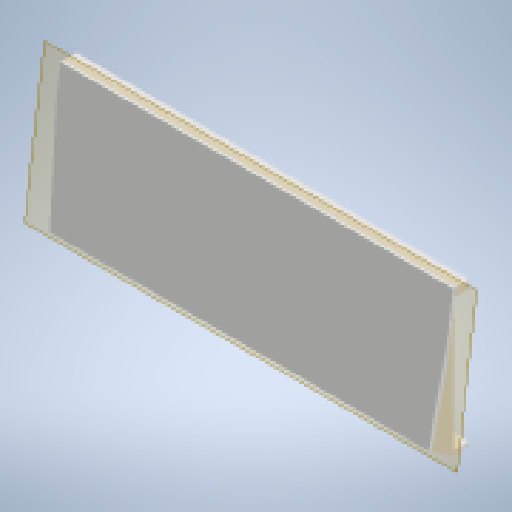
# Autodesk Inventor part: bottom
Saved by Autodesk Inventor 2024.2 (Build 282272000, 272)
## iProperties
Created: 2024-07-29
Part Number: bottom
Material: Generic
Document SubType Name: Modeling
Designer: Eric
Density: 1 g/cm^3
Appearance: Default
Author: Eric
Autodesk Inventor part; units mm, degrees
ref_plane "Work Plane1" through (0, 0, 9.8) normal (0, 0, 1) x (1, 0, 0)
sketch "Sketch1" plane through (0, 0, 9.8) normal (0, 0, 1) x (1, 0, 0)
  line L0 (145.35, 54.1) -> (-145.35, 54.1) projected
  line L1 (145.35, -54.1) -> (145.35, 54.1) projected
  line L2 (-145.35, -54.1) -> (145.35, -54.1) projected
  line L3 (-145.35, 54.1) -> (-145.35, -54.1) projected
  line L4 (143.1, 53.975) -> (-143.1, 53.975)
  line L5 (-143.1, 53.975) -> (-143.1, -51.85)
  line L6 (-143.1, -51.85) -> (143.1, -51.85)
  line L7 (143.1, -51.85) -> (143.1, 53.975)
  point P0 (0, 0)
  dimension "d0" = 0.125
  dimension "d1" = 2.25
  dimension "d2" = 2.25
  dimension "d3" = 2.25
  constraints: 8 end point, 2 parallel, 1 horizontal, 1 perpendicular
  measures "d0" distance between parallel lines of L0 L4
  measures "d1" distance between parallel lines of L2 L6
  measures "d2" distance between parallel lines of L1 L7
  measures "d3" distance between parallel lines of L3 L5
ref_plane "Work Plane2" through (-147.35, 31.7362, 13.0715) normal (0, 0.1305262, 0.9914449) x (1, 0, 0)
extrude "Extrusion1" add sketch "Sketch1" along normal up to surface contours L7 L6 L5 L4 surface through (-147.35, 31.7362, 13.0715) normal (0, 0.1305262, 0.9914449)
sketch "Sketch3" plane through (0, 0, 9.8) normal (0, 0, -1) x (-1, 0, 0)
  line L0 (143.1, 48.1) -> (-143.1, 48.1)
  line L1 (-143.1, -51.85) -> (-143.1, 53.975) projected
  line L2 (-143.1, -48.1) -> (143.1, -48.1)
  line L3 (143.1, 53.975) -> (143.1, -51.85) projected
  line L4 (-143.1, 53.975) -> (143.1, 53.975) projected
  line L5 (143.1, -51.85) -> (-143.1, -51.85) projected
  point P0 (0, 0)
  dimension "d8" = 5.875
  dimension "d9" = 3.75
  constraints: 4 end point, 3 point on line, 1 horizontal, 1 parallel
  measures "d8" distance between parallel lines of L4 L0
  measures "d9" distance between parallel lines of L5 L2
ref_plane "Work Plane3" through (-145.35, -54.1, -1.5) normal (0, 0, 1) x (1, 0, 0)
extrude "Extrusion2" add sketch "Sketch3" along normal up to surface (11.3 mm away) contours L0 L1 L4 L3 | L3 L5 L1 L2
sketch "Sketch4" plane through (-143.1, -48.1, 9.8) normal (-1, 0, 0) x (0, 0, 1)
  line L0 (14.2758, -3.75) -> (0.3437, 102.075) projected
  line L1 (13.3027, 3.6417) -> (1.7, -3.75)
  line L2 (-11.3, -3.75) -> (14.2758, -3.75) projected
  line L3 (0.7, -6) -> (0.7, -8) projected
  point P0 (-9.8, 48.1)
  dimension "d12" = 65
  dimension "d23" = 1
  constraints: 2 end point, 2 point on line
  measures "d12" angle of L0 L1
  measures "d23" distance from line of L3 L1.end
extrude "Extrusion3" cut sketch "Sketch4" against normal through all
sketch "Sketch5" plane through (-143.1, -51.85, -1.5) normal (0, -1, 0) x (1, 0, 0)
  line L0 (0, 13) -> (0, 24.6027) projected
  line L1 (0, 13) -> (5.4104, 24.6027)
  line L2 (0, 24.6027) -> (286.2, 24.6027) projected
  point P0 (143.1, 1.5)
  dimension "d15" = 65
  constraints: 2 end point, 1 point on line
  measures "d15" angle of L2 L1
sketch "Sketch6" plane through (-143.1, -48.1, 9.8) normal (-1, 0, 0) x (0, 0, 1)
  line L0 (1.7, -3.75) -> (3.3295, 79.3957)
  point P0 (-9.8, 48.1)
  point P1 (0.3437, 102.075)
  dimension "d16" = 22.875
  constraints: 2 end point
  measures "d16" distance of point (0.344, 102.075) L0.end
sweep "Sweep1" cut profiles "Sketch5" path "Sketch6"
mirror "Mirror1" about plane through (0, 0, 0) normal (1, 0, 0) of "Sweep1"
ref_plane "Work Plane4" through (-143.1, 53.7139, 8.1608) normal (0, 0.1305262, 0.9914449) x (1, 0, 0)
sketch "Sketch8" plane through (-143.1, 53.975, 10.1437) normal (0, 0.1305262, 0.9914449) x (1, 0, 0)
  line L0 (286.2, 0) -> (286.2, -22.875) projected
  line L1 (286.2, -15) -> (0, -15)
  line L2 (0, -22.875) -> (0, 0) projected
  line L3 (0, 0) -> (286.2, 0) projected
  point P0 (143.1, -52.1892)
  dimension "d20" = 15
  constraints: 2 end point, 2 point on line, 1 horizontal
  measures "d20" distance between parallel lines of L3 L1
extrude "Extrusion4" add sketch "Sketch8" against normal up to surface (2 mm away)
sketch "Sketch9" plane through (-143.1, -51.85, -1.5) normal (0, -1, 0) x (1, 0, 0)
  line L0 (286.2, 0) -> (286.2, 11.6437) projected
  line L1 (286.2, 3) -> (0, 3)
  line L2 (0, 10.3999) -> (0, 0) projected
  line L3 (286.2, 0) -> (0, 0) projected
  point P0 (143.1, 1.5)
  dimension "d24" = 3
  constraints: 2 end point, 2 point on line, 1 perpendicular
  measures "d24" distance between parallel lines of L3 L1
body "Solid1"
